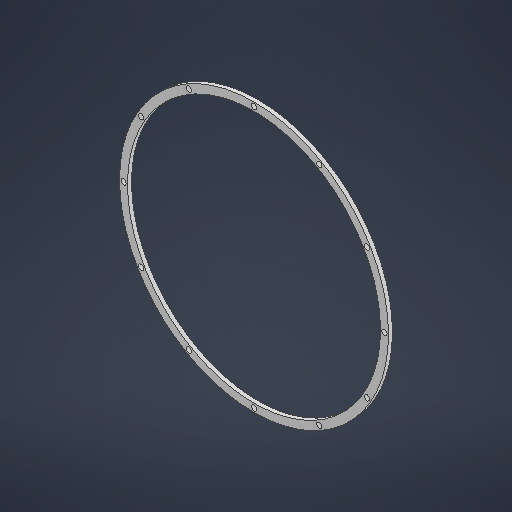
# Autodesk Inventor part: Aro del tambor
Saved by Autodesk Inventor 2026 (Build 300175050, 175E)
## iProperties
Created: 2025-07-12
Part Number: Aro del tambor
Material: Genérico
Document SubType Name: Modeling
Designer: Daniel Rodriguez
Density: 1 g/cm^3
Appearance: Valor por defecto
Author: Daniel Rodriguez
Autodesk Inventor part; units mm, degrees
ref_plane "YZ Plane" through (0, 0, 0) normal (1, 0, 0) x (0, 1, 0)
ref_plane "XZ Plane" through (0, 0, 0) normal (0, 1, 0) x (-1, 0, 0)
ref_plane "XY Plane" through (0, 0, 0) normal (0, 0, 1) x (1, 0, 0)
sketch "Boceto1" plane through (0, 0, 0) normal (0, 0, 1) x (1, 0, 0)
  circle A0 centre (0, 0) radius 337
  circle A1 centre (0, 0) radius 317
  dimension "d0" = 674
  dimension "d1" = 634
  constraints: 2 centre point, 2 coincident
  measures "d0" diameter of A0
  measures "d1" diameter of A1
extrude "Extrusión1" add sketch "Boceto1" along normal blind 10
sketch "Boceto2" plane through (0, 0, 10) normal (0, 0, 1) x (1, 0, 0)
  circle A0 centre (0, 0) radius 327 construction
  circle A1 centre (0, 0) radius 337 projected
  circle A2 centre (0, 327) radius 6.75
  circle A3 centre (-163.5, 283.1903) radius 6.75
  circle A4 centre (-283.1903, 163.5) radius 6.75
  circle A5 centre (-327, 0) radius 6.75
  circle A6 centre (-283.1903, -163.5) radius 6.75
  circle A7 centre (-163.5, -283.1903) radius 6.75
  circle A8 centre (0, -327) radius 6.75
  circle A9 centre (163.5, -283.1903) radius 6.75
  circle A10 centre (283.1903, -163.5) radius 6.75
  circle A11 centre (327, 0) radius 6.75
  circle A12 centre (283.1903, 163.5) radius 6.75
  circle A13 centre (163.5, 283.1903) radius 6.75
  dimension "d4" = 10
  dimension "d5" = 13.5
  dimension "d8" = 360
  constraints: 12 centre point, 1 coincident, 1 vertical alignment, 27 other
  measures "d5" diameter of A2
extrude "Extrusión2" cut sketch "Boceto2" against normal through all contours A2 | A3 | A4 | A5 | A6 | A7 | A8 | A9 | A10 | A11 | A12 | A13
